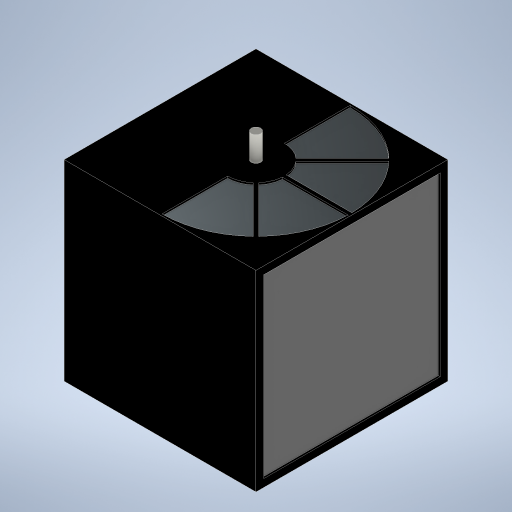
# Autodesk Inventor part: stepper_box
Saved by Autodesk Inventor 2024 (Build 280153000, 153)
## iProperties
Created: 2024-09-26
Part Number: stepper_box
Material: Generic
Document SubType Name: Modeling
Designer: skcre
Density: 1 g/cm^3
Appearance: Anodized - Black
Author: skcre
Autodesk Inventor part; units mm, degrees
ref_plane "YZ Plane" through (0, 0, 0) normal (1, 0, 0) x (0, 1, 0)
ref_plane "XZ Plane" through (0, 0, 0) normal (0, 1, 0) x (-1, 0, 0)
ref_plane "XY Plane" through (0, 0, 0) normal (0, 0, 1) x (1, 0, 0)
sketch "Sketch1" plane through (0, 0, 0) normal (0, 1, 0) x (-1, 0, 0)
  line L0 (-50, 50) -> (50, 50)
  line L1 (50, 50) -> (50, -50)
  line L2 (50, -50) -> (-50, -50)
  line L3 (-50, -50) -> (-50, 50)
  line L4 (-50, 50) -> (50, -50) construction
  line L5 (50, 50) -> (-50, -50) construction
  point P0 (0, 0)
  dimension "d0" = 100
  dimension "d1" = 100
  constraints: 12 end point, 2 midpoint, 2 parallel, 1 horizontal, 1 perpendicular
  measures "d0" distance of L1.end L2.end
  measures "d1" distance of L0.end L1.end
extrude "Extrusion1" add sketch "Sketch1" along normal blind 100
sketch "Sketch2" plane through (0, 100, 0) normal (0, 1, 0) x (1, 0, 0)
  line L0 (50, 50) -> (-50, 50) projected
  line L1 (-50, 50) -> (-50, -50) projected
  line L2 (-50, -50) -> (50, -50) projected
  line L3 (50, -50) -> (50, 50) projected
  line L4 (50, -50) -> (-50, 50)
  line L5 (-50, 50) -> (-50, -50) projected
  line L6 (-50, -50) -> (50, 50)
  circle A0 centre (0, 0) radius 2.5
  dimension "d4" = 5
  constraints: 4 end point, 1 centre point, 1 coincident, 1 perpendicular
  measures "d4" diameter of A0
extrude "Extrusion2" add sketch "Sketch2" along normal blind 13 contours A0 L4 L6 | L6 L4 A0 | L4 L6 A0 | A0 L6 L4
sketch "Sketch3" plane through (50, 0, 50) normal (1, 0, 0) x (0, 0, -1)
  line L0 (0, 0) -> (100, 0) projected
  line L1 (100, 0) -> (100, 100) projected
  line L2 (0, 100) -> (100, 100) projected
  line L3 (0, 0) -> (0, 100) projected
  line L4 (96, 96) -> (96, 4)
  line L5 (96, 4) -> (4, 4)
  line L6 (4, 4) -> (4, 96)
  line L7 (4, 96) -> (96, 96)
  point P0 (50, 0)
  dimension "d7" = 4
  constraints: 8 end point, 3 other
  measures "d7" distance between parallel lines of L2 L7
extrude "Extrusion3" cut sketch "Sketch3" against normal blind 1 contours L4 L5 L6 L7
sketch "Sketch4" plane through (0, 100, 0) normal (0, 1, 0) x (1, 0, 0)
  circle A0 centre (0, 0) radius 2.5 projected
  circle A1 centre (0, 0) radius 49
  circle A2 centre (0, 0) radius 14.7708
  line L0 (50, -50) -> (50, 50) projected
  line L1 (0, 0) -> (50, 50)
  line L2 (-50, -50) -> (50, -50) projected
  line L3 (0, 0) -> (50, -50)
  line L4 (0, -50) -> (0, 50)
  line L5 (50, 50) -> (-50, 50) projected
  line L6 (-1, -50) -> (-1, 50)
  line L7 (50.7071, -49.2929) -> (1.4142, 0)
  line L8 (1.4142, 0) -> (50.7071, 49.2929)
  line L9 (49.2929, -50.7071) -> (-1.4142, 0)
  line L10 (-1.4142, 0) -> (49.2929, 50.7071)
  line L11 (0, 0) -> (50, 0)
  line L12 (0, -1) -> (50, -1)
  line L13 (0, 1) -> (50, 1)
  point P0 (9.7134, 11.1276)
  point P1 (33.9339, 35.3481)
  point P2 (0, 49)
  point P3 (0, 14.7708)
  point P4 (14.7369, 1)
  point P5 (48.9898, 1)
  point P6 (35.3481, 33.9339)
  point P7 (11.1276, 9.7134)
  point P8 (33.9339, -35.3481)
  point P9 (9.7134, -11.1276)
  point P10 (0, -14.7708)
  point P11 (0, -49)
  point P12 (48.9898, -1)
  point P13 (14.7369, -1)
  point P14 (11.1276, -9.7134)
  point P15 (35.3481, -33.9339)
  dimension "d10" = 1
  dimension "d11" = 1
  dimension "d12" = 1
  dimension "d13" = 1
  dimension "d14" = 1
  constraints: 22 end point, 3 parallel, 2 centre point, 2 midpoint, 1 coincident, 1 perpendicular, 2 other
  measures "d10" distance between parallel lines of L4 L6
  measures "d11" distance between parallel lines of L3 L7
  measures "d12" distance between parallel lines of L3 L9
  measures "d13" distance between parallel lines of L11 L12
  measures "d14" distance between parallel lines of L11 L13
extrude "Extrusion4" cut sketch "Sketch4" against normal blind 1 contours A2 L8 A1 L13 | L12 A1 L7 A2 | A2 L4 A1 L10 | L9 A1 L4 A2
body "Solid1"
